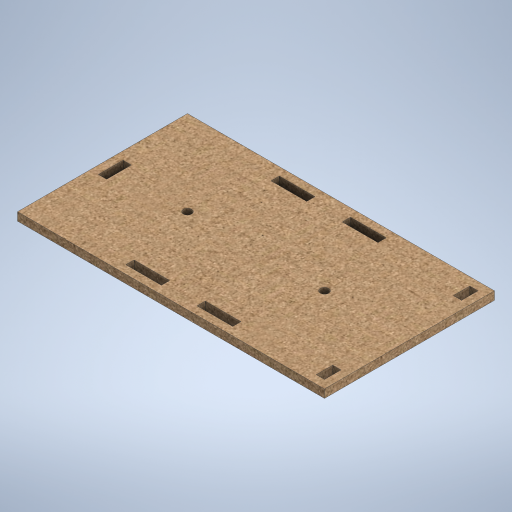
# Autodesk Inventor part: Case_Base2
Saved by Autodesk Inventor 2024 (Build 280153000, 153)
## iProperties
Created: 2023-11-23
Part Number: Case_Base2
Material: MDF Tablero de fibras de densidad media
Document SubType Name: Modeling
Designer: marco
Density: 0.8 g/cm^3
Appearance: Cartón - Ondulado
Author: marco
Autodesk Inventor part; units mm, degrees
ref_plane "YZ Plane" through (0, 0, 0) normal (1, 0, 0) x (0, 1, 0)
ref_plane "XZ Plane" through (0, 0, 0) normal (0, 1, 0) x (-1, 0, 0)
ref_plane "XY Plane" through (0, 0, 0) normal (0, 0, 1) x (1, 0, 0)
sketch "Boceto1" plane through (0, 0, 0) normal (0, 1, 0) x (-1, 0, 0)
  line L0 (-50, 28) -> (-53, 28)
  line L1 (-50, -28) -> (-50, -22)
  line L2 (-50, -28) -> (-53, -28)
  circle A0 centre (-25, 0) radius 1.5
  circle A1 centre (25, 0) radius 1.5
  line L3 (-53, -25) -> (-53, -28)
  line L4 (-53, -22) -> (-53, -25)
  line L5 (-50, -22) -> (-53, -22)
  line L6 (-50, -28) -> (-50, -22)
  line L7 (-53, -25) -> (-53, -28)
  line L8 (-53, -22) -> (-53, -25)
  line L9 (53, 4.5) -> (53, -4.5)
  line L10 (50, 4.5) -> (53, 4.5)
  line L11 (50, -4.5) -> (50, 4.5)
  line L12 (53, -4.5) -> (50, -4.5)
  line L13 (-50, 22) -> (-50, 28)
  line L14 (-53, 22) -> (-50, 22)
  line L15 (-53, 28) -> (-53, 22)
  line L16 (-50, 28) -> (-53, 28)
  line L17 (19.5, 28) -> (19.5, 25)
  line L18 (6.5, 28) -> (19.5, 28)
  line L19 (6.5, 25) -> (6.5, 28)
  line L20 (19.5, 25) -> (6.5, 25)
  line L21 (56, 31) -> (56, -31)
  line L22 (-56, 31) -> (56, 31)
  line L23 (-56, -31) -> (-56, 31)
  line L24 (56, -31) -> (-56, -31)
  line L25 (-19.5, 28) -> (-19.5, 25)
  line L26 (-6.5, 28) -> (-19.5, 28)
  line L27 (-6.5, 25) -> (-6.5, 28)
  line L28 (-19.5, 25) -> (-6.5, 25)
  line L29 (-19.5, -28) -> (-19.5, -25)
  line L30 (-6.5, -28) -> (-19.5, -28)
  line L31 (-6.5, -25) -> (-6.5, -28)
  line L32 (-19.5, -25) -> (-6.5, -25)
  line L33 (19.5, -25) -> (19.5, -28)
  line L34 (6.5, -25) -> (19.5, -25)
  line L35 (6.5, -28) -> (6.5, -25)
  line L36 (19.5, -28) -> (6.5, -28)
  constraints: 74 end point, 2 centre point
extrude "Extrusión1" add sketch "Boceto1" along normal blind 3
